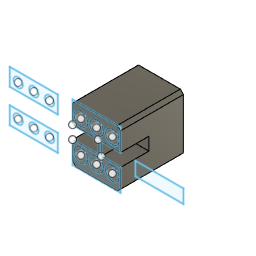
PartnerPDM Connector Rev2 (Autodesk Fusion 360 design; units mm, degrees)
Autodesk Fusion 360 part; units mm, degrees
sketch "Sketch1" plane through (0, 0, 0) normal (0, 1, 0) x (1, 0, 0)
  line L0 (0.6195, -2.3211) -> (15.9195, -2.3211)
  line L1 (15.9195, 15.7789) -> (0.6195, 15.7789)
  circle A0 centre (8.2695, 1.6789) radius 2.15
  line L2 (15.9195, 4.6789) -> (9.7695, 4.6789)
  line L3 (8.7695, 4.6789) -> (0.6195, 4.6789)
  line L4 (0.6195, 8.7789) -> (8.7695, 8.7789)
  line L5 (9.7695, 8.7789) -> (15.9195, 8.7789)
  circle A1 centre (13.2695, 1.6789) radius 2.15
  circle A2 centre (3.2695, 1.6789) radius 2.15
  circle A3 centre (8.2695, 11.7789) radius 2.15
  circle A4 centre (13.2695, 11.7789) radius 2.15
  circle A5 centre (3.2695, 11.7789) radius 2.15
  circle A6 centre (-6.7305, 1.6789) radius 1.45
  circle A7 centre (-11.7305, 1.6789) radius 1.45
  circle A8 centre (-16.7305, 1.6789) radius 1.45
  line L6 (-4.0805, -1.3211) -> (-19.3805, -1.3211)
  line L7 (-19.3805, -1.3211) -> (-19.3805, 4.1789)
  line L8 (-19.3805, 4.1789) -> (-4.0805, 4.1789)
  line L9 (-4.0805, 4.1789) -> (-4.0805, -1.3211)
  circle A9 centre (-6.7305, 11.7789) radius 1.45
  circle A10 centre (-16.7305, 11.7789) radius 1.45
  circle A11 centre (-11.7305, 11.7789) radius 1.45
  line L10 (-4.0805, 9.2789) -> (-19.3805, 9.2789)
  line L11 (-4.0805, 14.7789) -> (-4.0805, 9.2789)
  line L12 (-19.3805, 14.7789) -> (-4.0805, 14.7789)
  line L13 (-19.3805, 9.2789) -> (-19.3805, 14.7789)
  line L14 (20.6195, 4.5789) -> (35.9195, 4.5789)
  line L15 (35.9195, 4.5789) -> (35.9195, 8.8789)
  line L16 (35.9195, 8.8789) -> (20.6195, 8.8789)
  line L17 (20.6195, 8.8789) -> (20.6195, 4.5789)
  line L18 (9.7695, 8.7789) -> (9.7695, 4.6789)
  line L19 (8.7695, 4.6789) -> (8.7695, 8.7789)
  line L20 (15.9195, -2.3211) -> (15.9195, 4.6789)
  line L21 (0.6195, -2.3211) -> (0.6195, 4.6789)
  line L22 (15.9195, 8.7789) -> (15.9195, 15.7789)
  line L23 (0.6195, 15.7789) -> (0.6195, 8.7789)
  dimension "d2" = 7
  dimension "d4" = 7
  dimension "d7" = 4.3
  dimension "d8" = 4.3
  dimension "d9" = 4.3
  dimension "d10" = 5
  dimension "d11" = 5
  dimension "d12" = 4
  dimension "d14" = 4.3
  dimension "d15" = 4.3
  dimension "d16" = 4.3
  dimension "d17" = 5
  dimension "d18" = 5
  dimension "d21" = 2.9
  dimension "d22" = 2.9
  dimension "d23" = 2.9
  dimension "d25" = 5.5
  dimension "d29" = 5
  dimension "d30" = 5
  dimension "d34" = 2.9
  dimension "d35" = 2.9
  dimension "d36" = 2.9
  dimension "d38" = 5.5
  dimension "d39" = 5
  dimension "d40" = 5
  dimension "d49" = 4.3
  dimension "d50" = 15.3
  dimension "d77" = 4.1
  dimension "d80" = 20
  dimension "d81" = 15.3
  dimension "d84" = 7.65
  dimension "d85" = 7.65
  dimension "d86" = 7.65
  dimension "d87" = 7.65
  dimension "d88" = 15.3
  dimension "d89" = 20
  constraint horizontal L0
  constraint horizontal L2
  constraint coincident L3.start L2
  constraint collinear L2 L3
  constraint coincident L5.start L4
  constraint horizontal L10
  constraint vertical L13
  constraint horizontal L12
  constraint vertical L11
  constraint horizontal L14
  constraint vertical L15
  constraint horizontal L16
  constraint vertical L17
  constraint vertical L18
  constraint vertical L19
  constraint vertical L20
  constraint vertical L21
  constraint vertical L9
  constraint vertical L7
  measures "d2" distance of L3.end L0.start
  measures "d4" distance of L4.start L1.end
  measures "d7" diameter of A0
  measures "d8" diameter of A1
  measures "d9" diameter of A2
  measures "d10" distance of A0.centre A1.centre
  measures "d11" distance of A0.centre A2.centre
  measures "d12" distance of L0 A2.centre
  measures "d14" diameter of A3
  measures "d15" diameter of A4
  measures "d16" diameter of A5
  measures "d17" distance of A3.centre A4.centre
  measures "d18" distance of A5.centre A3.centre
  measures "d21" diameter of A6
  measures "d22" diameter of A7
  measures "d23" diameter of A8
  measures "d25" distance of L6.end L7.end
  measures "d29" distance of A7.centre A8.centre
  measures "d30" distance of A6.centre A7.centre
  measures "d34" diameter of A9
  measures "d35" diameter of A11
  measures "d36" diameter of A10
  measures "d38" distance of L10.end L12.start
  measures "d39" distance of A10.centre A11.centre
  measures "d40" distance of A9.centre A11.centre
  measures "d49" distance of L14.end L15.end
  measures "d50" distance of L14.start L14.end
  measures "d77" distance of L2.end L5.start
  measures "d80" distance of L14.end L20
  measures "d81" distance of L0.end L0.start
  measures "d84" distance of A7.centre L9
  measures "d85" distance of A7.centre L7
  measures "d86" horizontal distance of A11.centre L11.start
  measures "d87" horizontal distance of A11.centre L12.start
  measures "d88" distance of L7 L9
  measures "d89" distance of L6.end L21
combine "Combine1" [no effect]
move_body "Move6" [no effect]
extrude "Extrude7" add sketch "Sketch1" along normal blind 20 contours L0 L1 L2 L3 L4 L5 L18 L19 L20 L21 L22 L23 makes body 1
extrude "Extrude8" add sketch "Sketch1" along normal blind 2.7 separate body contours L6 L7 L8 L9 | L10 L11 L12 L13 makes body 2 at (-11.7667, 0, 0.8031) makes body 3 at (-11.7667, 0, -14.2609)
extrude "Extrude9" add sketch "Sketch1" along normal blind 11 separate body contours L14 L15 L16 L17 makes body 4
move_body "Move7" bodies 4 to x (1, 0, 0) y (0, 1, 0) z (0, 0, 1) at (0, 9, 0)
move_body "Move8" bodies 4 to x (1, 0, 0) y (0, 1, 0) z (0, 0, 1) at (-20, 0, 0)
combine "Combine2" operation add target body 4 tool bodies 1
move_body "Move9" bodies 3 2 to x (1, 0, 0) y (0, 1, 0) z (0, 0, 1) at (0, 8, 0)
move_body "Move10" bodies 3 2 to x (1, 0, 0) y (0, 1, 0) z (0, 0, 1) at (20, 0, 0)
chamfer "Chamfer1" distance 0.7 angle 45 1 edges at (1.9176, 10.7, -2.2032) on bodies 2
chamfer "Chamfer2" distance 0.7 angle 45 1 edges at (6.9176, 10.7, -2.2032) on bodies 2
chamfer "Chamfer3" distance 0.7 angle 45 1 edges at (11.9176, 10.7, -2.2032) on bodies 2
chamfer "Chamfer4" distance 0.7 angle 45 1 edges at (1.9176, 10.7, -12.3032) on bodies 3
chamfer "Chamfer5" distance 0.7 angle 45 1 edges at (6.9176, 10.7, -12.3032) on bodies 3
chamfer "Chamfer6" distance 0.7 angle 45 1 edges at (11.9176, 10.7, -12.3032) on bodies 3
combine "Combine3" operation add target body 3 tool bodies 2 4
chamfer "Chamfer7" distance 2 angle 45 1 edges at (0.6195, 10, 2.3211) on bodies 3
chamfer "Chamfer8" distance 2 angle 45 1 edges at (15.9195, 10, 2.3211) on bodies 3
chamfer "Chamfer9" distance 2 angle 45 1 edges at (0.6195, 10, -15.7789) on bodies 3
chamfer "Chamfer10" distance 2 angle 45 1 edges at (15.9195, 10, -15.7789) on bodies 3
delete_face "DeleteFace1" 1 faces at (14.5861, 6.6667, 1.6545) on bodies 3
chamfer "Chamfer11" distance 1 angle 45 1 edges at (15.9195, 10, 2.3211) on bodies 3
delete_face "DeleteFace2" 1 faces at (1.2861, 6.6667, 0.9878) on bodies 3
chamfer "Chamfer12" distance 1 angle 45 1 edges at (0.6195, 10, 2.3211) on bodies 3
delete_face "DeleteFace3" 1 faces at (14.5861, 6.6667, -15.1122) on bodies 3
chamfer "Chamfer13" distance 1 angle 45 1 edges at (15.9195, 10, -15.7789) on bodies 3
delete_face "DeleteFace4" 1 faces at (1.2861, 6.6667, -14.4455) on bodies 3
chamfer "Chamfer14" distance 1 angle 45 1 edges at (0.6195, 10, -15.7789) on bodies 3
